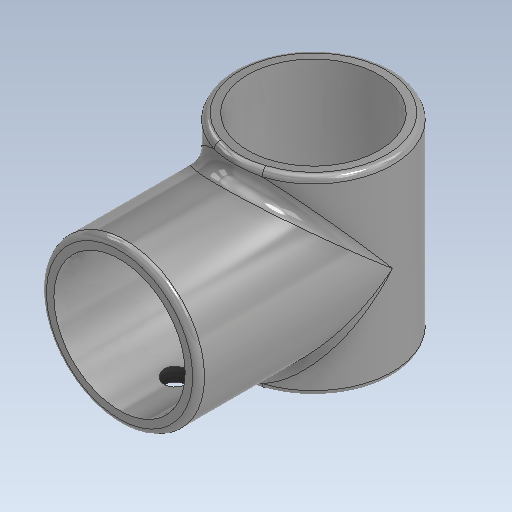
# Autodesk Inventor part: L10-7
Saved by Autodesk Inventor 2021 (Build 250183000, 183)
## iProperties
Created: 2020-04-23
Part Number: L10-7
Material: Aluminium Cast
Document SubType Name: Modeling
Designer: Hannah
Density: 3.0005 g/cm^3
Appearance: Aluminum - Dark
Mass: 200 g
Surface Area: 313.347 cm^2
Volume: 66.6556 cm^3
Catalog Web Link: https://keesystems.com/store/fittings/kee-lite/l10-single-socket-tee.html
Vendor: Kee Systems
Description: single socket tee
Size: 7
Author: Hannah
Revision Number: -
Autodesk Inventor part; units mm, degrees
ref_plane "XY Plane" through (0, 0, 0) normal (0, 0, 1) x (1, 0, 0)
sketch "Sketch1" plane through (0, 0, 0) normal (0, 0, 1) x (1, 0, 0)
  circle A0 centre (0, 0) radius 22
  circle A1 centre (0, 0) radius 26.5
  dimension "d1" = 53
  dimension "d2" = 44
  constraints: 2 centre point, 2 coincident
  measures "d1" diameter of A1
  measures "d2" diameter of A0
sketch "Sketch1 outline for Extrusion1" plane through (0, 0, 0) normal (0, 0, 1) x (1, 0, 0)
  circle A0 centre (0, 0) radius 26.5
extrude "Extrusion1" add sketch "Sketch1 outline for Extrusion1" along normal blind 65
sketch "Sketch2" plane through (0, 0, 0) normal (0, 1, 0) x (-1, 0, 0)
  circle A0 centre (0, 0) radius 22
  circle A1 centre (0, 0) radius 26.5
  dimension "d5" = 44
  dimension "d6" = 53
  constraints: 2 centre point, 2 coincident
  measures "d5" diameter of A0
  measures "d6" diameter of A1
sketch "Sketch2 outline for Extrusion2" plane through (0, 0, 0) normal (0, 1, 0) x (-1, 0, 0)
  circle A0 centre (0, 0) radius 26.5
extrude "Extrusion2" add sketch "Sketch2 outline for Extrusion2" along normal mid plane 64
sketch "Sketch2 outline for Extrusion3" plane through (0, 0, 0) normal (0, 1, 0) x (-1, 0, 0)
  circle A0 centre (0, 0) radius 22
extrude "Extrusion3" cut sketch "Sketch2 outline for Extrusion3" against normal up to surface (64 mm away) from surface at 32
sketch "Sketch1 outline for Extrusion4" plane through (0, 0, 0) normal (0, 0, 1) x (1, 0, 0)
  circle A0 centre (0, 0) radius 22
extrude "Extrusion4" cut sketch "Sketch1 outline for Extrusion4" along normal up to surface (65 mm away)
fillet "Fillet1" radius 5 2 edges at (0, 26.5, 26.5) (0, -26.5, 26.5)
hole "Hole1" at (0, 0, 0) direction (-1, 0, 0) diameter 8.376 end through all thread size "M10x1.5" class "6H" standard "ISO Metric profile"
ref_plane "Work Plane1" through (0, 0, 45.75) normal (0, 0, 1) x (1, 0, 0)
hole "Hole2" at (0, 0, 45.75) direction (0, -1, 0) diameter 8.376 end through all thread size "M10x1.5" class "6H" standard "ISO Metric profile"
fillet "Fillet2" radius 2 3 edges at (26.5, 32, 0) (-26.5, 0, 65) (26.5, -32, 0)
equation "\"d5\" = d2"
equation "\"d6\" = d1"
equation "\"d23\" = -0.5 * d3 + 0.25 * d1"
equation "\"d3\" = 65"
body "Solid1"
